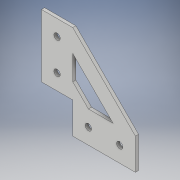
# Autodesk Inventor part: special brace
Saved by Autodesk Inventor 2018 (Build 220112000, 112)
## iProperties
Created: 2018-12-12
Part Number: special brace
Material: Generic
Document SubType Name: Modeling
Designer: s-4008082
Density: 1 g/cm^3
Appearance: Default
Author: s-4008082
Autodesk Inventor part; units mm, degrees
ref_plane "YZ Plane" through (0, 0, 0) normal (1, 0, 0) x (0, 1, 0)
ref_plane "XZ Plane" through (0, 0, 0) normal (0, 1, 0) x (-1, 0, 0)
ref_plane "XY Plane" through (0, 0, 0) normal (0, 0, 1) x (1, 0, 0)
sketch "Sketch1" plane through (0, 0, 0) normal (0, 0, 1) x (1, 0, 0)
  line L0 (0, 0) -> (25.4, 0)
  line L1 (25.4, 0) -> (25.4, 50.8)
  line L2 (25.4, 50.8) -> (0, 50.8)
  line L3 (0, 50.8) -> (0, 0)
  line L4 (25.4, 0) -> (76.2, 0)
  line L5 (76.2, 0) -> (76.2, -25.4)
  line L6 (76.2, -25.4) -> (25.4, -25.4)
  line L7 (25.4, -25.4) -> (25.4, 0)
  line L8 (76.2, 0) -> (25.4, 50.8)
  line L9 (25.4, 32.6931) -> (58.0931, 0)
  line L10 (25.4, 12.6979) -> (38.0979, 0)
  dimension "d0" = 25.4
  dimension "d1" = 50.8
  dimension "d2" = 50.8
  dimension "d3" = 25.4
  dimension "d21" = 45
  constraints: 22 end point, 4 parallel, 4 point on line, 2 horizontal, 2 perpendicular
  measures "d0" distance of L1.end L2.end
  measures "d1" distance of L0.end L1.end
  measures "d2" distance of L5.end L6.end
  measures "d3" distance of L4.end L5.end
  measures "d21" angle of L1 L9
extrude "Extrusion3" add sketch "Sketch1" along normal blind 2.54 contours L3 L2 L1 L0 | L1 L10 L4 | L4 L5 L6 L7 | L8 L4 L9 L1
sketch "Sketch3" plane through (0, 0, 2.54) normal (0, 0, 1) x (1, 0, 0)
  circle A0 centre (12.7, 12.7) radius 2.5797
  circle A1 centre (12.7, 38.1) radius 2.5797
  circle A2 centre (38.1, -12.7) radius 2.5797
  circle A3 centre (63.5, -12.7) radius 2.5797
  line L0 (25.4, 0) -> (25.4, -25.4) projected
  line L1 (25.4, -25.4) -> (76.2, -25.4) projected
  line L2 (76.2, -25.4) -> (76.2, 0) projected
  line L3 (0, 0) -> (25.4, 0) projected
  line L4 (0, 50.8) -> (0, 0) projected
  line L5 (25.4, 50.8) -> (0, 50.8) projected
  dimension "d26" = 12.7
  dimension "d27" = 12.7
  dimension "d28" = 12.7
  dimension "d29" = 12.7
  dimension "d30" = 12.7
  dimension "d31" = 12.7
  dimension "d32" = 12.7
  dimension "d33" = 12.7
  dimension "d34" = 5.1594
  dimension "d35" = 5.1594
  dimension "d36" = 5.1594
  dimension "d37" = 5.1594
  constraints: 4 centre point
  measures "d26" distance from line of L0 A2.centre
  measures "d27" distance from line of L1 A2.centre
  measures "d28" distance from line of L2 A3.centre
  measures "d29" distance from line of L1 A3.centre
  measures "d30" distance from line of L3 A0.centre
  measures "d31" distance from line of L4 A0.centre
  measures "d32" distance from line of L4 A1.centre
  measures "d33" distance from line of L5 A1.centre
  measures "d34" diameter of A1
  measures "d35" diameter of A0
  measures "d36" diameter of A2
  measures "d37" diameter of A3
extrude "Extrusion5" cut sketch "Sketch3" against normal blind 2.54
body "Solid1"
